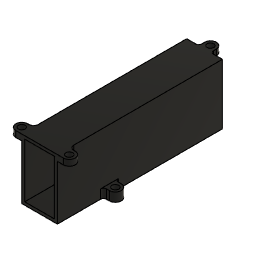
バッテリーケース (Autodesk Fusion 360 design; units mm, degrees)
Autodesk Fusion 360 part; units mm, degrees
sketch "スケッチ1" plane through (0, 0, 0) normal (0, 0, 1) x (1, 0, 0)
  line L0 (0, 0) -> (24, 0)
  line L1 (24, 0) -> (24, 111)
  line L2 (24, 111) -> (0, 111)
  line L3 (0, 111) -> (0, 0)
  dimension "d1" = 24
  dimension "d2" = 111
  constraint horizontal L0
  constraint vertical L1
  constraint horizontal L2
  constraint vertical L3
  constraint coincident L0.start L3.end
  measures "d1" distance of L0.start L0.end
  measures "d2" distance of L0.start L2.end
extrude "押し出し1" add sketch "スケッチ1" along normal blind 38
sketch "スケッチ2" plane through (0, 0, 0) normal (0, -1, 0) x (1, 0, 0)
  line L0 (0, 0) -> (24, 0)
  line L1 (24, 0) -> (24, 38)
  line L2 (24, 38) -> (0, 38)
  line L3 (0, 38) -> (0, 0)
  line L4 (2, 36) -> (22, 36)
  line L5 (22, 36) -> (22, 2)
  line L6 (22, 2) -> (2, 2)
  line L7 (2, 2) -> (2, 36)
  constraint horizontal L4
  constraint vertical L5
  constraint horizontal L6
  constraint vertical L7
extrude "押し出し2" cut sketch "スケッチ2" against normal blind 109 contours L4 L5 L6 L7
sketch "スケッチ3" plane through (0, 0, 38) normal (0, 0, 1) x (-1, 0, 0)
  line L0 (0, -111) -> (0, 0)
  line L1 (0, 0) -> (-24, 0)
  line L2 (-24, 0) -> (-24, -111)
  line L3 (-24, -111) -> (0, -111)
sketch "スケッチ4" plane through (0, 0, 0) normal (0, 0, -1) x (1, 0, 0)
  line L0 (0, 0) -> (0, -111)
  line L1 (0, -111) -> (24, -111)
  line L2 (24, -111) -> (24, 0)
  line L3 (24, 0) -> (0, 0)
  line L4 (12, -35) -> (28, -35)
  line L5 (12, -35) -> (-4, -35)
  circle A0 centre (-4, -35) radius 1.75
  circle A1 centre (28, -35) radius 1.75
  circle A2 centre (28, -35) radius 4
  circle A3 centre (-4, -35) radius 4
  line L6 (-4, -31) -> (0, -31)
  line L7 (28, -31) -> (24, -31)
  line L8 (28, -39) -> (24, -39)
  line L9 (-4, -39) -> (0, -39)
  dimension "d10" = 3.5
  dimension "d11" = 3.5
  constraint horizontal L4
  constraint parallel L4 L5
  constraint coincident L5.end A0.centre
  constraint coincident L4.end A1.centre
  constraint concentric A1 A2
  constraint concentric A0 A3
  constraint tangent L0 A3
  constraint coincident A3 L6.start
  constraint coincident L0 L6.end
  constraint tangent A3 L6
  constraint perpendicular L0 L6
  constraint coincident A2 L7.start
  constraint coincident L2 L7.end
  constraint tangent A2 L7
  constraint perpendicular L2 L7
  constraint coincident A2 L8.start
  constraint coincident L2 L8.end
  constraint tangent A2 L8
  constraint perpendicular L2 L8
  constraint coincident A3 L9.start
  constraint coincident L0 L9.end
  constraint tangent A3 L9
  constraint perpendicular L0 L9
  measures "d10" diameter of A0
  measures "d11" diameter of A1
extrude "押し出し3" add sketch "スケッチ4" against normal blind 5 contours L0 A3 L6 | A3 | L0 A3 L9 | L2 A2 L7 | L2 A2 L8 | A2
fillet "フィレット1" radius 2 4 edges at (24, 31, 2.5) (24, 39, 2.5) (0, 39, 2.5) (0, 31, 2.5)
sketch "スケッチ5" plane through (0, 0, 38) normal (0, 0, 1) x (-1, 0, 0)
  line L0 (-12, 0) -> (4, 0)
  line L1 (4, 0) -> (4, -4)
  circle A0 centre (4, -4) radius 1.75
  circle A1 centre (4, -4) radius 4
  line L2 (-12, 0) -> (-28, 0)
  line L3 (-28, 0) -> (-28, -4)
  circle A2 centre (-28, -4) radius 1.75
  circle A3 centre (-28, -4) radius 4
  line L4 (-28, -8) -> (-24, -8)
  line L5 (4, -8) -> (0, -8)
  line L6 (4, 0) -> (-1.5, 0)
  line L7 (4, -8) -> (-1, -8)
  line L8 (-28, -8) -> (-23.7099, -8)
  line L9 (-28, 0) -> (-23.351, 0)
  line L10 (0, -8) -> (0, 0)
  line L11 (-24, -8) -> (-24, 0)
  dimension "d16" = 3.5
  dimension "d17" = 3.5
  constraint horizontal L0
  constraint perpendicular L0 L1
  constraint coincident L1.end A0.centre
  constraint concentric A0 A1
  constraint parallel L0 L2
  constraint perpendicular L2 L3
  constraint coincident L3.end A2.centre
  constraint concentric A2 A3
  constraint coincident A3 L4.start
  constraint tangent A3 L4
  constraint horizontal L4
  constraint coincident A1 L5.start
  constraint tangent A1 L5
  constraint parallel L4 L5
  constraint coincident L0 L6.end
  constraint tangent A1 L6
  constraint tangent A1 L7
  constraint tangent A3 L8
  constraint coincident L2 L9.end
  constraint tangent A3 L9
  constraint coincident L10.end origin
  constraint perpendicular L0 L10
  constraint coincident L9 L11.end
  measures "d16" diameter of A0
  measures "d17" diameter of A2
extrude "押し出し4" add sketch "スケッチ5" against normal blind 4.5
sketch "スケッチ6" plane through (0, 0, 38) normal (0, 0, 1) x (-1, 0, 0)
  line L0 (-12, -111) -> (-12, -115)
  circle A0 centre (-12, -115) radius 1.75
  circle A1 centre (-12, -115) radius 4
  line L1 (-8, -115) -> (-8, -111)
  line L2 (-16, -115) -> (-16, -111)
  line L3 (-16, -111) -> (-8, -111)
  dimension "d20" = 3.5
  constraint vertical L0
  constraint coincident L0.end A0.centre
  constraint concentric A0 A1
  constraint coincident A1 L1.start
  constraint tangent A1 L1
  constraint parallel L0 L1
  constraint coincident A1 L2.start
  constraint tangent A1 L2
  constraint parallel L1 L2
  constraint perpendicular L1 L3
  measures "d20" diameter of A0
extrude "押し出し5" add sketch "スケッチ6" against normal blind 4.5
fillet "フィレット2" radius 2 2 edges at (8, 111, 35.75) (16, 111, 35.75)
fillet "フィレット3" radius 3 2 edges at (24, 8, 35.75) (0, 8, 35.75)
extrude "押し出し6" add sketch "スケッチ3" 1 faces at (10.0949, 44.3401, 38) along normal blind 0.5
extrude "押し出し7" cut 1 faces at (8.6667, 72.6667, 36) along direction (0, 0, 1) blind 0.5
extrude "押し出し8" cut 1 faces at (10.0949, 44.3401, 38.5) along direction (0, 0, -1) blind 1
extrude "押し出し9" add 1 faces at (8.6667, 72.6667, 36.5) along direction (0, 0, -1) blind 1
extrude "押し出し10" add 1 faces at (8, 64.3333, 0) along direction (0, 0, -1) blind 1
extrude "押し出し11" cut 1 faces at (15.3333, 72.6667, 2) along direction (0, 0, -1) blind 1
sketch "スケッチ7" plane through (0, 0, 37.5) normal (0, 0, 1) x (-1, 0, 0)
  circle A0 centre (-28, -4) radius 1.75
  circle A1 centre (-12, -115) radius 1.75
  circle A2 centre (4, -4) radius 1.75
  line L0 (-24, -111) -> (-18, -111)
  arc A3 (-16, -113) -> (-18, -111) centre (-18, -113) ccw
  line L1 (-16, -113) -> (-16, -115)
  arc A4 (-16, -115) -> (-8, -115) centre (-12, -115) ccw
  line L2 (-8, -115) -> (-8, -113)
  arc A5 (-6, -111) -> (-8, -113) centre (-6, -113) ccw
  line L3 (-6, -111) -> (0, -111)
  line L4 (0, -111) -> (0, -11)
  arc A6 (3, -8) -> (0, -11) centre (3, -11) ccw
  line L5 (3, -8) -> (4, -8)
  arc A7 (4, -8) -> (4, 0) centre (4, -4) ccw
  line L6 (4, 0) -> (-28, 0)
  arc A8 (-28, 0) -> (-28, -8) centre (-28, -4) ccw
  line L7 (-28, -8) -> (-27, -8)
  arc A9 (-24, -11) -> (-27, -8) centre (-27, -11) ccw
  line L8 (-24, -11) -> (-24, -111)
  circle A10 centre (-12, -115) radius 2.25
  circle A11 centre (-28, -4) radius 2.25
  circle A12 centre (4, -4) radius 2.25
  dimension "d39" = 4.5
  dimension "d40" = 4.5
  dimension "d41" = 4.5
  constraint concentric A1 A10
  constraint concentric A0 A11
  constraint concentric A2 A12
  measures "d39" diameter of A10
  measures "d40" diameter of A11
  measures "d41" diameter of A12
extrude "押し出し12" cut sketch "スケッチ7" against normal blind 8 contours A10 | A11 | A12
sketch "スケッチ8" plane through (0, 0, 5) normal (0, 0, 1) x (-1, 0, 0)
  circle A0 centre (4, -35) radius 1.75
  arc A1 (4, -39) -> (4, -31) centre (4, -35) ccw
  line L0 (4, -31) -> (2, -31)
  arc A2 (0, -29) -> (2, -31) centre (2, -29) ccw
  line L1 (0, -29) -> (0, -41)
  arc A3 (2, -39) -> (0, -41) centre (2, -41) ccw
  line L2 (2, -39) -> (4, -39)
  circle A4 centre (4, -35) radius 2.25
  dimension "d44" = 4.5
  constraint concentric A0 A4
  measures "d44" diameter of A4
extrude "押し出し13" cut sketch "スケッチ8" against normal blind 25 contours A4
sketch "スケッチ9" plane through (0, 0, 5) normal (0, 0, 1) x (-1, 0, 0)
  circle A0 centre (-28, -35) radius 1.75
  line L0 (-26, -31) -> (-28, -31)
  arc A1 (-28, -31) -> (-28, -39) centre (-28, -35) ccw
  line L1 (-28, -39) -> (-26, -39)
  arc A2 (-24, -41) -> (-26, -39) centre (-26, -41) ccw
  line L2 (-24, -41) -> (-24, -29)
  arc A3 (-26, -31) -> (-24, -29) centre (-26, -29) ccw
  circle A4 centre (-28, -35) radius 2.25
  dimension "d47" = 4.5
  constraint concentric A0 A4
  measures "d47" diameter of A4
extrude "押し出し14" cut sketch "スケッチ9" against normal blind 13 contours A4
sketch "スケッチ10" plane through (0, 0, -1) normal (0, 0, -1) x (1, 0, 0)
  circle A0 centre (28, -35) radius 2.25
  circle A1 centre (-4, -35) radius 2.25
  line L0 (0, -41) -> (0, -111)
  line L1 (0, -111) -> (24, -111)
  line L2 (24, -111) -> (24, -41)
  arc A2 (26, -39) -> (24, -41) centre (26, -41) ccw
  line L3 (26, -39) -> (28, -39)
  arc A3 (28, -39) -> (28, -31) centre (28, -35) ccw
  line L4 (28, -31) -> (26, -31)
  arc A4 (24, -29) -> (26, -31) centre (26, -29) ccw
  line L5 (24, -29) -> (24, 0)
  line L6 (24, 0) -> (0, 0)
  line L7 (0, 0) -> (0, -29)
  arc A5 (-2, -31) -> (0, -29) centre (-2, -29) ccw
  line L8 (-2, -31) -> (-4, -31)
  arc A6 (-4, -31) -> (-4, -39) centre (-4, -35) ccw
  line L9 (-4, -39) -> (-2, -39)
  arc A7 (0, -41) -> (-2, -39) centre (-2, -41) ccw
  line L10 (-4, -31) -> (28, -31)
  line L11 (28, -39) -> (-4, -39)
  line L12 (0, -31) -> (0, -39)
  line L13 (24, -31) -> (24, -39)
  constraint coincident L8.end A6.start
  constraint coincident A3.end L4.start
  constraint coincident L3.end A3.start
  constraint coincident A6.end L9.start
  constraint coincident L10 L12.start
  constraint coincident L11 L12.end
  constraint perpendicular L11 L12
  constraint coincident L10 L13.start
  constraint coincident L11 L13.end
  constraint perpendicular L11 L13
extrude "押し出し15" add sketch "スケッチ10" along normal blind 2 contours L8 A6 L9 L10 L11 L12 | L3 A3 L4 L10 L11 L13
sketch "スケッチ11" plane through (0, 0, -3) normal (0, 0, -1) x (1, 0, 0)
  circle A0 centre (-4, -35) radius 2.25
  arc A1 (-4, -31) -> (-4, -39) centre (-4, -35) ccw
  line L0 (-4, -39) -> (0, -39)
  line L1 (0, -39) -> (0, -31)
  line L2 (0, -31) -> (-4, -31)
  circle A2 centre (-4, -35) radius 4
  constraint concentric A0 A2
extrude "押し出し16" cut sketch "スケッチ11" against normal blind 2 contours L1 L2 A2 | L0 L1 A2
sketch "スケッチ12" plane through (0, 0, -3) normal (0, 0, -1) x (1, 0, 0)
  circle A0 centre (28, -35) radius 2.25
  line L0 (28, -31) -> (24, -31)
  line L1 (24, -31) -> (24, -39)
  line L2 (24, -39) -> (28, -39)
  arc A1 (28, -39) -> (28, -31) centre (28, -35) ccw
  circle A2 centre (28, -35) radius 4
  constraint concentric A0 A2
extrude "押し出し17" cut sketch "スケッチ12" against normal blind 2 contours L0 L1 A2 | L1 L2 A2
extrude "押し出し18" add 1 faces at (8, 87.6667, -1) along direction (0, 0, -1) blind 2
extrude "押し出し19" cut 1 faces at (15.3333, 72.6667, 1) along direction (0, 0, -1) blind 2
extrude "押し出し20" cut 1 faces at (24.5833, 35, 5) along direction (0, 0, -1) blind 2
extrude "押し出し21" cut 1 faces at (-0.795, 35, 5) along direction (0, 0, -1) blind 2
